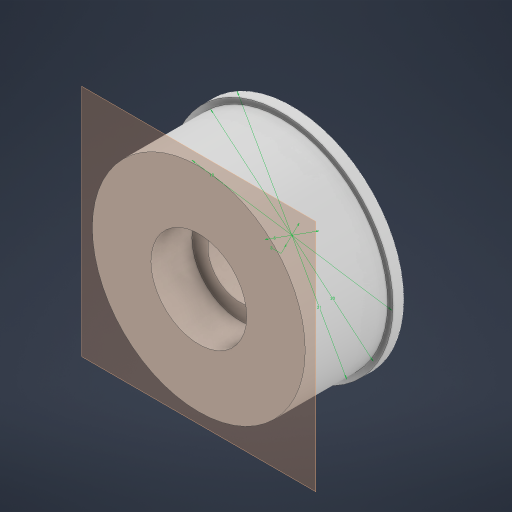
# Autodesk Inventor part: wheel
Saved by Autodesk Inventor 2023 (Build 270158000, 158)
## iProperties
Created: 2023-12-13
Part Number: wheel
Material: 一般
Document SubType Name: Modeling
Designer: IshiiLabHonda
Density: 1 g/cm^3
Appearance: 既定
Author: IshiiLabHonda
Autodesk Inventor part; units mm, degrees
ref_plane "YZ Plane" through (0, 0, 0) normal (1, 0, 0) x (0, 1, 0)
ref_plane "XZ Plane" through (0, 0, 0) normal (0, 1, 0) x (-1, 0, 0)
ref_plane "XY Plane" through (0, 0, 0) normal (0, 0, 1) x (1, 0, 0)
sketch "スケッチ1" plane through (0, 0, 0) normal (0, 0, 1) x (1, 0, 0)
  circle A0 centre (0, 0) radius 10 construction
  circle A1 centre (0, 0) radius 10.5 construction
  circle A2 centre (0, 0) radius 3 construction
  circle A3 centre (0, 0) radius 9.5 construction
  circle A4 centre (0, 0) radius 1.5
  dimension "d0" = 20
  dimension "d1" = 21
  dimension "d2" = 6
  dimension "d3" = 19
  dimension "d10" = 3
  constraints: 5 centre point, 5 coincident
  measures "d0" diameter of A0
  measures "d1" diameter of A1
  measures "d2" diameter of A2
  measures "d3" diameter of A3
  measures "d10" diameter of A4
sketch "スケッチ2" plane through (0, 0, 0) normal (0, 0, 1) x (1, 0, 0)
  circle A0 centre (0, 0) radius 9.5 construction
  circle A1 centre (0, 0) radius 10 construction
  circle A2 centre (0, 0) radius 9.5
  circle A3 centre (0, 0) radius 10
  constraints: 2 centre point, 2 coincident, 2 concentric
extrude "押し出し1" add sketch "スケッチ2" along normal blind 8.75
sketch "スケッチ4" plane through (0, 0, 0) normal (0, 0, 1) x (1, 0, 0)
  circle A0 centre (0, 0) radius 3 construction
  circle A1 centre (0, 0) radius 9.5 construction
  circle A2 centre (0, 0) radius 9.5
  circle A3 centre (0, 0) radius 10 projected
  circle A4 centre (0, 0) radius 3
  constraints: 2 centre point, 2 coincident, 1 concentric
extrude "押し出し3" add sketch "スケッチ4" along normal blind 8.75 contours A2 | A4
sketch "スケッチ6" plane through (0, 0, 0) normal (0, 0, 1) x (1, 0, 0)
  circle A0 centre (0, 0) radius 10 construction
  circle A1 centre (0, 0) radius 10.5 construction
  circle A2 centre (0, 0) radius 3 construction
  circle A3 centre (0, 0) radius 9.5 construction
  circle A4 centre (0, 0) radius 1.5
  circle A5 centre (0, 0) radius 10.5
  circle A6 centre (0, 0) radius 10
  circle A7 centre (0, 0) radius 10 projected
  circle A8 centre (0, 0) radius 9.5
  circle A9 centre (0, 0) radius 3
  dimension "d15" = 20
  dimension "d16" = 21
  dimension "d17" = 6
  dimension "d18" = 19
  dimension "d19" = 3
  constraints: 9 centre point, 9 coincident, 4 concentric
  measures "d15" diameter of A0
  measures "d16" diameter of A1
  measures "d17" diameter of A2
  measures "d18" diameter of A3
  measures "d19" diameter of A4
extrude "押し出し6" add sketch "スケッチ6" along normal blind 1 contours A5
sketch "スケッチ7" plane through (0, 0, 0) normal (0, 0, 1) x (1, 0, 0)
  circle A0 centre (0, 0) radius 10 construction
  circle A1 centre (0, 0) radius 10.5 construction
  circle A2 centre (0, 0) radius 3 construction
  circle A3 centre (0, 0) radius 9.5 construction
  circle A4 centre (0, 0) radius 1.5
  circle A5 centre (0, 0) radius 10.5
  circle A6 centre (0, 0) radius 10
  circle A7 centre (0, 0) radius 9.5
  circle A8 centre (0, 0) radius 3
  circle A9 centre (0, 0) radius 4
  dimension "d22" = 20
  dimension "d23" = 21
  dimension "d24" = 6
  dimension "d25" = 19
  dimension "d26" = 3
  dimension "d27" = 8
  constraints: 10 centre point, 9 coincident, 4 concentric
  measures "d22" diameter of A0
  measures "d23" diameter of A1
  measures "d24" diameter of A2
  measures "d25" diameter of A3
  measures "d26" diameter of A4
  measures "d27" diameter of A9
extrude "押し出し7" add sketch "スケッチ7" against normal blind 2 contours A9
sketch "スケッチ8" plane through (0, 0, 0) normal (0, 0, 1) x (1, 0, 0)
  circle A0 centre (0, 0) radius 10 construction
  circle A1 centre (0, 0) radius 10.5 construction
  circle A2 centre (0, 0) radius 3 construction
  circle A3 centre (0, 0) radius 9.5 construction
  circle A4 centre (0, 0) radius 1.5
  circle A5 centre (0, 0) radius 10.5
  circle A6 centre (0, 0) radius 10
  circle A7 centre (0, 0) radius 9.5
  circle A8 centre (0, 0) radius 3
  circle A9 centre (0, 0) radius 4
  dimension "d30" = 20
  dimension "d31" = 21
  dimension "d32" = 6
  dimension "d33" = 19
  dimension "d34" = 3
  dimension "d35" = 8
  constraints: 10 centre point, 9 coincident, 4 concentric
  measures "d30" diameter of A0
  measures "d31" diameter of A1
  measures "d32" diameter of A2
  measures "d33" diameter of A3
  measures "d34" diameter of A4
  measures "d35" diameter of A9
extrude "押し出し8" cut sketch "スケッチ8" along normal blind 20 contours A4
sketch "スケッチ9" plane through (0, 0, 0) normal (0, 0, 1) x (1, 0, 0)
  circle A0 centre (0, 0) radius 10 construction
  circle A1 centre (0, 0) radius 10.5 construction
  circle A2 centre (0, 0) radius 3 construction
  circle A3 centre (0, 0) radius 9.5 construction
  circle A4 centre (0, 0) radius 1.5
  circle A5 centre (0, 0) radius 10.5
  circle A6 centre (0, 0) radius 10
  circle A7 centre (0, 0) radius 9.5
  circle A8 centre (0, 0) radius 3
  circle A9 centre (0, 0) radius 4
  dimension "d38" = 20
  dimension "d39" = 21
  dimension "d40" = 6
  dimension "d41" = 19
  dimension "d42" = 3
  dimension "d43" = 8
  constraints: 10 centre point, 9 coincident, 4 concentric
  measures "d38" diameter of A0
  measures "d39" diameter of A1
  measures "d40" diameter of A2
  measures "d41" diameter of A3
  measures "d42" diameter of A4
  measures "d43" diameter of A9
extrude "押し出し9" cut sketch "スケッチ9" along normal blind 20 contours A8
ref_plane "作業平面1" through (0, 0, 8.75) normal (0, 0, 1) x (1, 0, 0)
sketch "スケッチ10" plane through (0, 0, 8.75) normal (0, 0, 1) x (1, 0, 0)
  circle A0 centre (0, 0) radius 4.5
  dimension "d47" = 9
  constraints: 1 centre point, 1 coincident
  measures "d47" diameter of A0
extrude "押し出し10" cut sketch "スケッチ10" against normal blind 3.85
